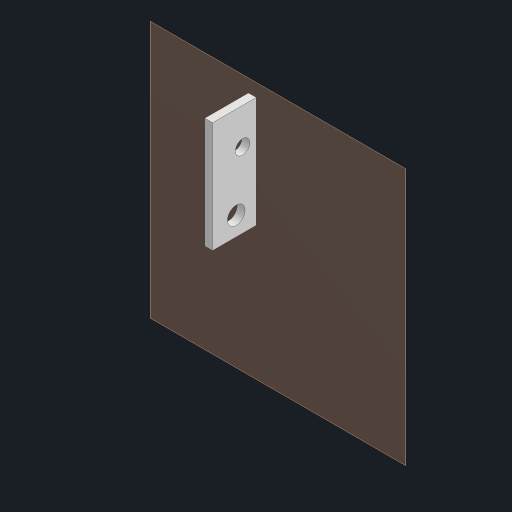
# Autodesk Inventor part: right_gear_holder
Saved by Autodesk Inventor 2023 (Build 270158000, 158)
## iProperties
Created: 2024-04-23
Part Number: right_gear_holder
Material: Generic
Document SubType Name: Modeling
Designer: szymo
Density: 1 g/cm^3
Appearance: Default
Author: szymo
Autodesk Inventor part; units mm, degrees
ref_plane "YZ Plane" through (0, 0, 0) normal (1, 0, 0) x (0, 1, 0)
ref_plane "XZ Plane" through (0, 0, 0) normal (0, 1, 0) x (-1, 0, 0)
ref_plane "XY Plane" through (0, 0, 0) normal (0, 0, 1) x (1, 0, 0)
ref_plane "Work Plane1" through (0, 0, 0) normal (0, 0, 1) x (1, 0, 0)
sketch "Sketch1" plane through (0, 0, 0) normal (0, 0, 1) x (1, 0, 0)
  line L0 (23.5, 88.5) -> (-23.5, 88.5) projected
  line L1 (-23.5, 88.5) -> (-23.5, 36.5) projected
  line L2 (-26.5, 33.5) -> (-89, 33.5) projected
  line L3 (-89, 33.5) -> (-89, -72.5) projected
  line L4 (-89, -72.5) -> (-77, -72.5) projected
  line L5 (-74, -75.5) -> (-74, -93.5) projected
  line L6 (-74, -93.5) -> (74, -93.5) projected
  line L7 (74, -93.5) -> (74, -75.5) projected
  line L8 (77, -72.5) -> (89, -72.5) projected
  line L9 (89, -72.5) -> (89, 33.5) projected
  line L10 (89, 33.5) -> (26.5, 33.5) projected
  line L11 (23.5, 36.5) -> (23.5, 88.5) projected
  line L12 (-4.5, 81.5) -> (-4.5, 36.5) projected
  line L13 (-7.5, 33.5) -> (-13.5, 33.5) projected
  line L14 (-16.5, 36.5) -> (-16.5, 81.5) projected
  line L15 (-13.5, 84.5) -> (-7.5, 84.5) projected
  line L16 (16.5, 81.5) -> (16.5, 36.5) projected
  line L17 (13.5, 33.5) -> (7.5, 33.5) projected
  line L18 (4.5, 36.5) -> (4.5, 81.5) projected
  line L19 (7.5, 84.5) -> (13.5, 84.5) projected
  line L20 (-16.5, 88.5) -> (-22.5, 88.5)
  line L21 (-22.5, 88.5) -> (-22.5, 3.75)
  line L22 (-22.5, 3.75) -> (-16.5, 3.75)
  line L23 (-16.5, 3.75) -> (-16.5, 88.5)
  line L24 (-32.2, 4.75) -> (-59.9, 4.75)
  arc A0 (13.5, 33.5) -> (16.5, 36.5) centre (13.5, 36.5) ccw projected
  arc A1 (4.5, 36.5) -> (7.5, 33.5) centre (7.5, 36.5) ccw projected
  arc A2 (7.5, 84.5) -> (4.5, 81.5) centre (7.5, 81.5) ccw projected
  arc A3 (16.5, 81.5) -> (13.5, 84.5) centre (13.5, 81.5) ccw projected
  arc A4 (-4.5, 81.5) -> (-7.5, 84.5) centre (-7.5, 81.5) ccw projected
  arc A5 (-7.5, 33.5) -> (-4.5, 36.5) centre (-7.5, 36.5) ccw projected
  arc A6 (-16.5, 36.5) -> (-13.5, 33.5) centre (-13.5, 36.5) ccw projected
  arc A7 (-13.5, 84.5) -> (-16.5, 81.5) centre (-13.5, 81.5) ccw projected
  arc A8 (-26.5, 33.5) -> (-23.5, 36.5) centre (-26.5, 36.5) ccw projected
  arc A9 (-74, -75.5) -> (-77, -72.5) centre (-77, -75.5) ccw projected
  arc A10 (77, -72.5) -> (74, -75.5) centre (77, -75.5) ccw projected
  arc A11 (23.5, 36.5) -> (26.5, 33.5) centre (26.5, 36.5) ccw projected
  point P0 (0, 0)
  point P1 (-16.5, 36.5)
  point P2 (-16.5, 81.5)
  dimension "d0" = 1
  dimension "d2" = 1
  constraints: 10 end point, 2 horizontal, 2 parallel, 1 collinear, 1 perpendicular, 1 point on line, 2 other
  measures "d0" distance between parallel lines of L1 L21
  measures "d2" distance between parallel lines of L24 L22
ref_plane "Work Plane2" through (-89, -40.3889, 33.5) normal (0, 0, 1) x (1, 0, 0)
extrude "Extrusion1" add sketch "Sketch1" along normal up to surface (33.5 mm away) contours L23 L14 L22 L21 L0
sketch "Sketch2" plane through (-22.5, 3.75, 0) normal (-1, 0, 0) x (0, 0, 1)
  arc A0 (13.7043, 8.7757) -> (14.863, 10.545) centre (10.3771, 12.2188) ccw projected
  arc A1 (14.863, 10.545) -> (15.4685, 10.512) centre (15.375, 14.375) ccw projected
  arc A2 (15.4685, 10.512) -> (16.4285, 8.6275) centre (20.1095, 11.6893) ccw projected
  arc A3 (16.4285, 8.6275) -> (17.3146, 8.863) centre (15.375, 14.375) ccw projected
  arc A4 (17.3146, 8.863) -> (17.2121, 10.9755) centre (12.599, 9.6929) ccw projected
  arc A5 (17.2121, 10.9755) -> (17.7212, 11.3047) centre (15.375, 14.375) ccw projected
  arc A6 (17.7212, 11.3047) -> (19.6056, 10.3444) centre (20.7839, 14.9851) ccw projected
  arc A7 (19.6056, 10.3444) -> (20.184, 11.0558) centre (15.375, 14.375) ccw projected
  arc A8 (20.184, 11.0558) -> (18.8594, 12.7045) centre (15.8813, 8.9554) ccw projected
  arc A9 (18.8594, 12.7045) -> (19.0778, 13.2702) centre (15.375, 14.375) ccw projected
  arc A10 (19.0778, 13.2702) -> (21.1668, 13.6008) centre (19.3923, 18.0479) ccw projected
  arc A11 (21.1668, 13.6008) -> (21.2166, 14.5164) centre (15.375, 14.375) ccw projected
  arc A12 (21.2166, 14.5164) -> (19.1758, 15.0716) centre (18.9701, 10.288) ccw projected
  arc A13 (19.1758, 15.0716) -> (19.02, 15.6576) centre (15.375, 14.375) ccw projected
  arc A14 (19.02, 15.6576) -> (20.5157, 17.153) centre (16.4662, 19.7077) ccw projected
  arc A15 (20.5157, 17.153) -> (20.0178, 17.923) centre (15.375, 14.375) ccw projected
  arc A16 (20.0178, 17.923) -> (18.0404, 17.1726) centre (20.6858, 13.1817) ccw projected
  arc A17 (18.0404, 17.1726) -> (17.57, 17.5552) centre (15.375, 14.375) ccw projected
  arc A18 (17.57, 17.5552) -> (17.9011, 19.644) centre (13.1233, 19.3306) ccw projected
  arc A19 (17.9011, 19.644) -> (17.0457, 19.9743) centre (15.375, 14.375) ccw projected
  arc A20 (17.0457, 19.9743) -> (15.887, 18.205) centre (20.3729, 16.5312) ccw projected
  arc A21 (15.887, 18.205) -> (15.2815, 18.238) centre (15.375, 14.375) ccw projected
  arc A22 (15.2815, 18.238) -> (14.3215, 20.1225) centre (10.6405, 17.0607) ccw projected
  arc A23 (14.3215, 20.1225) -> (13.4354, 19.887) centre (15.375, 14.375) ccw projected
  arc A24 (13.4354, 19.887) -> (13.5379, 17.7745) centre (18.151, 19.0571) ccw projected
  arc A25 (13.5379, 17.7745) -> (13.0288, 17.4453) centre (15.375, 14.375) ccw projected
  arc A26 (13.0288, 17.4453) -> (11.1444, 18.4056) centre (9.9661, 13.7649) ccw projected
  arc A27 (11.1444, 18.4056) -> (10.566, 17.6942) centre (15.375, 14.375) ccw projected
  arc A28 (10.566, 17.6942) -> (11.8906, 16.0455) centre (14.8687, 19.7946) ccw projected
  arc A29 (11.8906, 16.0455) -> (11.6722, 15.4798) centre (15.375, 14.375) ccw projected
  arc A30 (11.6722, 15.4798) -> (9.5832, 15.1492) centre (11.3577, 10.7021) ccw projected
  arc A31 (9.5832, 15.1492) -> (9.5334, 14.2336) centre (15.375, 14.375) ccw projected
  arc A32 (9.5334, 14.2336) -> (11.5742, 13.6784) centre (11.7799, 18.462) ccw projected
  arc A33 (11.5742, 13.6784) -> (11.73, 13.0924) centre (15.375, 14.375) ccw projected
  arc A34 (11.73, 13.0924) -> (10.2343, 11.597) centre (14.2838, 9.0423) ccw projected
  arc A35 (10.2343, 11.597) -> (10.7322, 10.827) centre (15.375, 14.375) ccw projected
  arc A36 (10.7322, 10.827) -> (12.7096, 11.5774) centre (10.0642, 15.5683) ccw projected
  arc A37 (12.7096, 11.5774) -> (13.18, 11.1948) centre (15.375, 14.375) ccw projected
  arc A38 (13.18, 11.1948) -> (12.8489, 9.106) centre (17.6267, 9.4194) ccw projected
  arc A39 (12.8489, 9.106) -> (13.7043, 8.7757) centre (15.375, 14.375) ccw projected
  circle A40 centre (15.375, 14.375) radius 6.75
  circle A41 centre (15.375, 14.375) radius 5.8433
  line L0 (21.2183, 14.375) -> (22.125, 14.375)
  circle A42 centre (10.5, 57.25) radius 5.5 projected
  point P0 (0, -3.75)
  dimension "d6" = 13.5
  dimension "d5" = 0.9067
  dimension "d9" = 11
  constraints: 3 horizontal, 2 coincident, 2 end point, 2 horizontal alignment, 5 other
  measures "d5" distance of L0.start L0.end
  measures "d9" diameter of A42
extrude "Extrusion2" cut sketch "Sketch2" against normal up to next contours A39 A38 A37 A36 A35 A34 A33 A32 A31 A30 A29 A28 A27 A26 A25 A24 A23 A22 A21 A20 A19 A18 A17 A16 A15 A14 A13 A12 A11 A10 A9 A8 A7 A6 A5 A4 A3 A2 A1 A0 | A0 A1 A2 A41 | A41 A36 A37 A38 | A4 A5 A6 A41 | A41 A32 A33 A34 | A8 A9 A10 A41 | A41 A28 A29 A30 | A41 A24 A25 A26 | A12 A13 A14 A41 | A41 A20 A21 A22 | A16 A17 A18 A41 | A40 | A42
body "Solid1"
